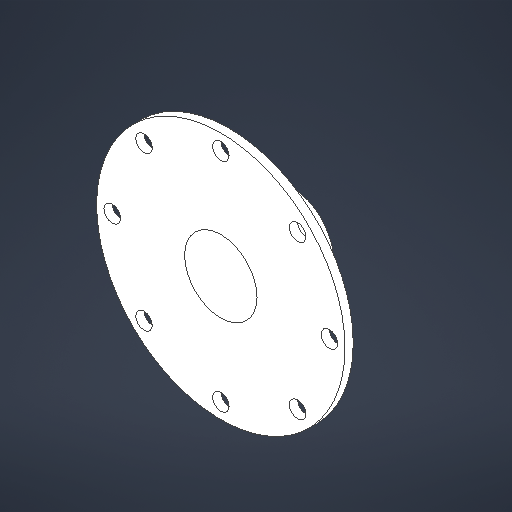
# Autodesk Inventor part: CESTO MEDIDOR ESPORAS
Saved by Autodesk Inventor 2026.2 (Build 302298000, 298)
## iProperties
Created: 2026-01-02
Part Number: CESTO MEDIDOR ESPORAS
Material: Genérico
Document SubType Name: Modeling
Designer: vicho
Density: 1 g/cm^3
Appearance: Valor por defecto
Author: vicho
Autodesk Inventor part; units mm, degrees
ref_plane "YZ Plane" through (0, 0, 0) normal (1, 0, 0) x (0, 1, 0)
ref_plane "XZ Plane" through (0, 0, 0) normal (0, 1, 0) x (-1, 0, 0)
ref_plane "XY Plane" through (0, 0, 0) normal (0, 0, 1) x (1, 0, 0)
sketch "Boceto1" plane through (0, 0, 0) normal (0, 0, 1) x (1, 0, 0)
  circle A0 centre (0, 0) radius 60
  circle A1 centre (0, 0) radius 48.5 construction
  circle A2 centre (0, 0) radius 52.5 construction
  line L0 (0, -61.2439) -> (0, 59.6068) construction
  line L1 (-77.557, 0) -> (94.8903, 0) construction
  circle A3 centre (0, 52.5) radius 4
  circle A4 centre (-37.1231, 37.1231) radius 4
  circle A5 centre (-52.5, 0) radius 4
  circle A6 centre (-37.1231, -37.1231) radius 4
  circle A7 centre (0, -52.5) radius 4
  circle A8 centre (37.1231, -37.1231) radius 4
  circle A9 centre (52.5, 0) radius 4
  circle A10 centre (37.1231, 37.1231) radius 4
  dimension "d2" = 105
  dimension "d0" = 120
  dimension "d1" = 97
  dimension "d3" = 8
  dimension "d6" = 360
  constraints: 10 centre point, 4 end point, 3 coincident, 3 point on line, 1 horizontal, 1 vertical, 1 vertical alignment, 19 other
  measures "d0" diameter of A0
  measures "d1" diameter of A1
  measures "d3" diameter of A3
extrude "Extrusión1" add sketch "Boceto1" along normal blind 4
sketch "Boceto2" plane through (0, 0, 0) normal (0, 0, -1) x (-1, 0, 0)
  circle A0 centre (0, 0) radius 20.5
  dimension "d10" = 41
  constraints: 1 centre point, 1 coincident
  measures "d10" diameter of A0
extrude "Extrusión2" add sketch "Boceto2" along normal blind 30
sketch "Boceto3" plane through (0, 0, -30) normal (0, 0, -1) x (-1, 0, 0)
  circle A0 centre (0, 0) radius 17.5
  dimension "d13" = 35
  constraints: 1 centre point, 1 coincident
  measures "d13" diameter of A0
extrude "Extrusión3" cut sketch "Boceto3" against normal blind 35
